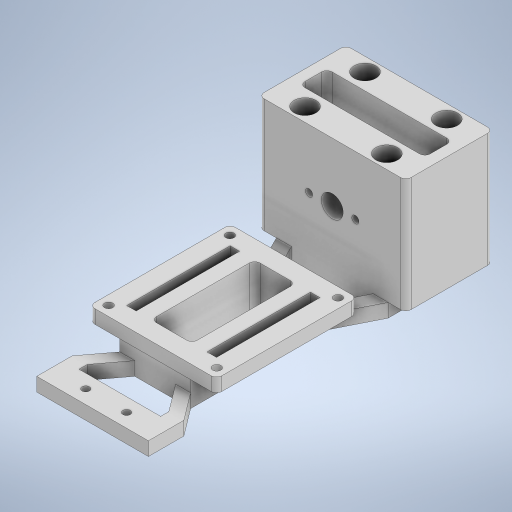
# Autodesk Inventor part: Houder encodere
Saved by Autodesk Inventor 2023 (Build 270158000, 158)
## iProperties
Created: 2023-03-09
Part Number: Houder encodere
Material: Generic
Document SubType Name: Modeling
Designer: daanj
Density: 1 g/cm^3
Appearance: Default
Author: daanj
Autodesk Inventor part; units mm, degrees
ref_plane "YZ Plane" through (0, 0, 0) normal (1, 0, 0) x (0, 1, 0)
ref_plane "XZ Plane" through (0, 0, 0) normal (0, 1, 0) x (-1, 0, 0)
ref_plane "XY Plane" through (0, 0, 0) normal (0, 0, 1) x (1, 0, 0)
sketch "Sketch1" plane through (0, 0, 0) normal (0, 1, 0) x (-1, 0, 0)
  line L0 (20.5, -60) -> (-20.5, -60)
  line L1 (-20.5, -60) -> (-20.5, 60)
  line L2 (-20.5, 60) -> (20.5, 60)
  line L3 (20.5, -60) -> (-20.5, 60) construction
  line L4 (-20.5, -60) -> (20.5, 60) construction
  circle A0 centre (7.5, 55) radius 1.35
  circle A1 centre (-7.5, 55) radius 1.35
  circle A2 centre (15, -33) radius 1.35
  circle A3 centre (15, -55) radius 1.35
  circle A4 centre (-15, -55) radius 1.35
  circle A5 centre (-15, -33) radius 1.35
  line L5 (-13, -13) -> (-13, 37)
  line L6 (13, 37) -> (13, -13)
  line L7 (20.5, -33) -> (20.5, -28)
  line L8 (20.5, -28) -> (13, -13)
  line L9 (-13, -13) -> (-20.5, -28)
  line L10 (20.5, 55) -> (20.5, 54)
  line L11 (20.5, 47) -> (13, 37)
  line L12 (-13, 37) -> (-20.5, 47)
  line L13 (20.5, 60) -> (20.5, 47)
  line L14 (20.5, -28) -> (20.5, -60)
  line L15 (16.5, -49) -> (-16.5, -49)
  line L16 (-16.5, -49) -> (-16.5, -39)
  line L17 (-16.5, -39) -> (16.5, -39)
  line L18 (16.5, -39) -> (16.5, -49)
  line L19 (15, -28) -> (-15, -28)
  line L20 (-15, -28) -> (-7.5, -13)
  line L21 (-7.5, -13) -> (7.5, -13)
  line L22 (7.5, -13) -> (15, -28)
  line L23 (7.5, -7) -> (-7.5, -7)
  line L24 (-7.5, -7) -> (-7.5, 31)
  line L25 (-7.5, 31) -> (7.5, 31)
  line L26 (7.5, 31) -> (7.5, -7)
  line L27 (7.5, 37) -> (-7.5, 37)
  line L28 (-7.5, 37) -> (-15, 47)
  line L29 (7.5, 37) -> (15, 47)
  line L30 (15, 47) -> (15, 50)
  line L31 (15, 50) -> (-15, 50)
  line L32 (-15, 50) -> (-15, 47)
  point P0 (0, 0)
  dimension "d0" = 41
  dimension "d1" = 120
  dimension "d2" = 5
  dimension "d3" = 2.7
  dimension "d5" = 22
  dimension "d6" = 15
  dimension "d7" = 7.5
  dimension "d8" = 30
  dimension "d9" = 15
  dimension "d10" = 88
  dimension "d11" = 50
  dimension "d12" = 26
  dimension "d14" = 13
  dimension "d15" = 5
  dimension "d16" = 8
  dimension "d17" = 33
  dimension "d18" = 16.5
  dimension "d19" = 10
  dimension "d20" = 6
  dimension "d21" = 5
  dimension "d22" = 15
  dimension "d23" = 6
  dimension "d25" = 6
  dimension "d28" = 5.5
  dimension "d29" = 5.5
  dimension "d30" = 5
  dimension "d33" = 0
  dimension "d34" = 5.5
  dimension "d35" = 5.5
  constraints: 66 end point, 9 parallel, 6 centre point, 5 equal radius, 5 horizontal, 5 perpendicular, 5 point on line, 3 horizontal alignment, 2 midpoint, 2 vertical alignment, 1 vertical
  measures "d0" distance of L0.start L0.end
  measures "d1" distance of L0.end L1.end
  measures "d2" distance from line of L2 A0.centre
  measures "d3" diameter of A0
  measures "d5" distance of A3.centre A2.centre
  measures "d6" distance of A1.centre A0.centre
  measures "d7" horizontal distance of point (0, 0) A0.centre
  measures "d8" distance of A5.centre A2.centre
  measures "d9" horizontal distance of point (0, 0) A2.centre
  measures "d10" vertical distance of A0.centre A2.centre
  measures "d11" distance of L5.start L5.end
  measures "d12" distance of L6.end L5.start
  measures "d14" distance from line of point (0, 0) L5
  measures "d15" distance of L7.start L7.end
  measures "d16" distance of L10.start L11.start
  measures "d17" distance of L15.start L15.end
  measures "d18" distance from line of point (0, 0) L18
  measures "d19" distance of L17.end L15.start
  measures "d20" distance from line of A3.centre L15
  measures "d21" distance of A2.centre L19.start
  measures "d22" distance of L20.end L21.end
  measures "d23" distance between parallel lines of L21 L23
  measures "d25" distance from line of L25 L6.start
  measures "d28" distance of L27.start L6.start
  measures "d29" distance of L12.end L28.end
  measures "d30" distance from line of L31 A0.centre
  measures "d33" vertical distance of L21.end L6.end
  measures "d34" distance of L6.end L21.end
  measures "d35" distance of L5.start L20.end
extrude "Extrusion1" add sketch "Sketch1" along normal blind 5 contours L0 L1 L9 L5 L12 L2 L13 L10 L11 L6 L8 L7 L14
sketch "Sketch2" plane through (0, 5, 0) normal (0, 1, 0) x (1, 0, 0)
  line L0 (-7.5, 13) -> (-15, 28) projected
  line L1 (-20.5, 28) -> (-15, 28)
  line L2 (15, 28) -> (7.5, 13) projected
  line L3 (13, 13) -> (20.5, 28) projected
  line L4 (15, 28) -> (20.5, 28)
  line L5 (20.5, 60) -> (-20.5, 60) projected
  line L6 (16.5, 39) -> (-16.5, 39) projected
  line L7 (-15, 28) -> (15, 28) projected
  circle A0 centre (-15, 33) radius 1.35 projected
  circle A1 centre (15, 33) radius 1.35 projected
  line L8 (-16.5, 49) -> (16.5, 49) projected
  circle A2 centre (15, 55) radius 1.35 projected
  circle A3 centre (-15, 55) radius 1.35 projected
  circle A4 centre (-15, 55) radius 4
  circle A5 centre (15, 55) radius 4
  circle A6 centre (15, 33) radius 4
  circle A7 centre (-15, 33) radius 4
  line L9 (-27, 60) -> (27, 60)
  line L10 (27, 60) -> (27, 28)
  line L11 (27, 28) -> (-27, 28)
  line L12 (-27, 28) -> (-27, 60)
  line L13 (-23, 49) -> (23, 49)
  line L14 (23, 49) -> (23, 39)
  line L15 (23, 39) -> (-23, 39)
  line L16 (-23, 39) -> (-23, 49)
  point P0 (0, 0)
  point P1 (0, 60)
  point P2 (0, 60)
  point P3 (0, 39)
  point P4 (0, 39)
  dimension "d36" = 8
  dimension "d37" = 8
  dimension "d38" = 8
  dimension "d39" = 8
  dimension "d90" = 54
  dimension "d91" = 46
  constraints: 20 end point, 6 coincident, 4 centre point, 4 horizontal, 4 midpoint, 4 parallel, 2 perpendicular, 1 point on line
  measures "d36" diameter of A4
  measures "d37" diameter of A5
  measures "d38" diameter of A6
  measures "d39" diameter of A7
  measures "d90" distance of L9.start L9.end
  measures "d91" distance of L14.end L15.end
extrude "Extrusion2" add sketch "Sketch2" along normal blind 42 contours L11 L12 L9 L5 L10 L4 L7 L1
sketch "Sketch3" plane through (-15, 0, -28) normal (0, 0, 1) x (1, 0, 0)
  line L0 (-5.5, 5) -> (-5.5, 47) projected
  line L1 (42, 47) -> (-12, 47) projected
  point P0 (15, 0)
  point P1 (15, 25.35)
  point P2 (35.5, 47)
  dimension "d42" = 20.5
  dimension "d43" = 21.65
  measures "d42" distance from line of L0 point (15, 25.35)
  measures "d43" distance from line of L1 point (15, 25.35)
hole "Hole1" at (0, 25.35, -28) direction (0, 0, -1) diameter 8 end through all
sketch "Sketch4" plane through (0, 5, 0) normal (0, 1, 0) x (1, 0, 0)
  line L0 (-7.5, -31) -> (-7.5, 7) projected
  line L1 (7.5, 7) -> (7.5, -31) projected
  line L2 (-7.5, 7) -> (7.5, 7) projected
  line L3 (7.5, -31) -> (-7.5, -31) projected
  line L4 (13, -37) -> (13, 13) projected
  line L5 (-13, 13) -> (13, 13)
  line L6 (13, 13) -> (13, -37)
  line L7 (13, -37) -> (-13, -37)
  line L8 (-13, -37) -> (-13, 13)
  point P0 (0, 0)
  constraints: 8 end point, 2 parallel, 1 horizontal, 1 perpendicular
extrude "Extrusion5" add sketch "Sketch4" along normal blind 5
sketch "Sketch6" plane through (-15, 0, -28) normal (0, 0, 1) x (1, 0, 0)
  circle A0 centre (15, 25.35) radius 4 projected
  circle A1 centre (15, 25.35) radius 8.5 construction
  line L0 (15, 25.35) -> (25.2915, 25.35) construction
  line L1 (26, 47) -> (26, 5) construction
  line L2 (25.2915, 25.35) -> (5.5322, 25.35) construction
  circle A2 centre (23.5, 25.35) radius 1.3
  circle A3 centre (6.5, 25.35) radius 1.3
  point P0 (15, 0)
  dimension "d70" = 17
  dimension "d71" = 2.6
  dimension "d72" = 2.6
  constraints: 4 end point, 3 centre point, 3 point on line, 2 point on circle, 1 coincident, 1 perpendicular
  measures "d70" diameter of A1
  measures "d71" diameter of A2
  measures "d72" diameter of A3
extrude "Extrusion6" cut sketch "Sketch6" against normal blind 10 contours A2 | A3
sketch "Sketch7" plane through (0, 10, 0) normal (0, 1, 0) x (1, 0, 0)
  line L0 (-23.3, 13.8) -> (23.3, 13.8)
  line L1 (23.3, 13.8) -> (23.3, -37.8)
  line L2 (23.3, -37.8) -> (-23.3, -37.8)
  line L3 (-23.3, -37.8) -> (-23.3, 13.8)
  circle A0 centre (-19.85, 10.25) radius 1.5
  circle A1 centre (19.85, 10.25) radius 1.5
  circle A2 centre (19.85, -34.25) radius 1.5
  circle A3 centre (-19.85, -34.25) radius 1.5
  line L4 (13, 13) -> (13, -37) projected
  line L5 (-7.5, 7) -> (-7.5, -31) projected
  line L6 (7.5, -31) -> (7.5, 7) projected
  line L7 (-7.5, 7) -> (7.5, 7)
  line L8 (7.5, 7) -> (7.5, -31)
  line L9 (7.5, -31) -> (-7.5, -31)
  line L10 (-7.5, -31) -> (-7.5, 7)
  line L11 (-13, 13) -> (-13, -37) projected
  line L12 (-13, 7) -> (-16.5, 7)
  line L13 (-16.5, 7) -> (-16.5, -31)
  line L14 (-16.5, -31) -> (-13, -31)
  line L15 (-13, -31) -> (-13, 7)
  line L16 (13, -37) -> (13, 13) projected
  line L17 (13, -31) -> (16.5, -31)
  line L18 (16.5, -31) -> (16.5, 7)
  line L19 (16.5, 7) -> (13, 7)
  line L20 (13, 7) -> (13, -31)
  point P0 (0, 0)
  point P1 (13, -12)
  point P2 (23.3, -12)
  dimension "d75" = 46.6
  dimension "d76" = 51.6
  dimension "d77" = 3
  dimension "d78" = 3
  dimension "d79" = 3
  dimension "d80" = 3
  dimension "d81" = 39.7
  dimension "d82" = 44.5
  dimension "d83" = 3.55
  dimension "d84" = 3.45
  dimension "d85" = 23.3
  dimension "d86" = 3.5
  dimension "d87" = 3.5
  constraints: 32 end point, 8 parallel, 6 point on line, 4 centre point, 4 horizontal, 4 perpendicular, 3 horizontal alignment, 2 midpoint, 2 vertical alignment
  measures "d75" distance of L1.end L2.end
  measures "d76" distance of L0.end L1.end
  measures "d77" diameter of A0
  measures "d78" diameter of A1
  measures "d79" diameter of A2
  measures "d80" diameter of A3
  measures "d81" distance of A1.centre A0.centre
  measures "d82" distance of A3.centre A0.centre
  measures "d83" distance from line of L0 A1.centre
  measures "d84" distance from line of L3 A0.centre
  measures "d85" distance from line of point (0, 0) L3
  measures "d86" distance of L14.end L13.end
  measures "d87" distance of L19.end L18.end
extrude "Extrusion7" add sketch "Sketch7" along normal blind 5
fillet "Fillet1" radius 2 16 edges at (-27, 26, -28) (27, 26, -28) (-23, 26, -39) (-27, 26, -60) (27, 26, -60) (23, 26, -49) (23, 26, -39) (-23, 26, -49) (-23.3, 12.5, -13.8) (-23.3, 12.5, 37.8) (23.3, 12.5, 37.8) (23.3, 12.5, -13.8) (-7.5, 7.5, -7) (-7.5, 7.5, 31) (7.5, 7.5, -7) (7.5, 7.5, 31)
body "Solid1"
